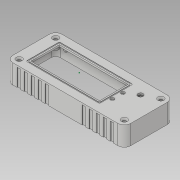
# Autodesk Inventor part: CAJA ELECTRONICA
Saved by Autodesk Inventor 2019 (Build 230136000, 136)
## iProperties
Created: 2020-02-13
Part Number: CAJA ELECTRONICA
Material: Genérico
Document SubType Name: Modeling
Designer: Luis Pujol
Density: 1 g/cm^3
Appearance: Valor por defecto
Author: Luis Pujol
## iProperties of the stored document TAPA SUPERIOR DOSF CO2_3DPrint.ipt
Created: 2020-02-13
Part Number: TAPA SUPERIOR DOSF CO2_3DPrint
Material: Genérico
Document SubType Name: Modeling
Designer: Luis Pujol
Density: 1 g/cm^3
Appearance: Valor por defecto
Author: Luis Pujol
Autodesk Inventor part; units mm, degrees
ref_plane "XZ Plane" through (0, 0, 0) normal (0, 1, 0) x (-1, 0, 0)
ref_plane "XY Plane" through (0, 0, 0) normal (0, 0, 1) x (1, 0, 0)
sketch "Boceto1" plane through (0, 0, 0) normal (0, 1, 0) x (-1, 0, 0)
  line L0 (48.8, 20.25) -> (-48.8, 20.25)
  line L1 (-48.8, 20.25) -> (-48.8, -20.25)
  line L2 (-48.8, -20.25) -> (48.8, -20.25)
  line L3 (48.8, -20.25) -> (48.8, 20.25)
  line L4 (48.8, 20.25) -> (-48.8, -20.25) construction
  line L5 (-48.8, 20.25) -> (48.8, -20.25) construction
  line L6 (-98.8, 35) -> (68.8, 35)
  line L7 (68.8, 35) -> (68.8, -35)
  line L8 (68.8, -35) -> (-98.8, -35)
  line L9 (-98.8, -35) -> (-98.8, 35)
  point P0 (0, 0)
  point P1 (0, 0)
  dimension "d5" = 97.6
  dimension "d6" = 40.5
  dimension "d7" = 70
  dimension "d8" = 20
  dimension "d9" = 50
  constraints: 20 end point, 4 parallel, 3 midpoint, 2 horizontal, 2 perpendicular
  measures "d5" distance of L2.end L1.end
  measures "d6" distance of L1.end L0.end
  measures "d7" distance of L6.end L7.end
  measures "d8" distance between parallel lines of L3 L7
  measures "d9" distance between parallel lines of L1 L9
extrude "Extrusión1" add sketch "Boceto1" along normal blind 2.5
sketch "Boceto2" plane through (0, 0, 0) normal (0, -1, 0) x (1, 0, 0)
  line L0 (-48.8, -20.25) -> (-48.8, 20.25) projected
  line L1 (-48.8, 20.25) -> (48.8, 20.25) projected
  line L2 (48.8, 20.25) -> (48.8, -20.25) projected
  line L3 (48.8, -20.25) -> (-48.8, -20.25) projected
  line L4 (98.8, 35) -> (-68.8, 35) projected
  line L5 (-68.8, 35) -> (-68.8, -35) projected
  line L6 (-68.8, -35) -> (98.8, -35) projected
  line L7 (98.8, -35) -> (98.8, 35) projected
  line L8 (46.5, 27.5) -> (-46.5, 27.5) construction
  line L9 (-46.5, 27.5) -> (-46.5, -27.5) construction
  line L10 (-46.5, -27.5) -> (46.5, -27.5) construction
  line L11 (46.5, -27.5) -> (46.5, 27.5) construction
  line L12 (46.5, 27.5) -> (-46.5, -27.5) construction
  line L13 (-46.5, 27.5) -> (46.5, -27.5) construction
  circle A0 centre (46.5, -27.5) radius 3
  circle A1 centre (-46.5, -27.5) radius 3
  circle A2 centre (46.5, 27.5) radius 3
  circle A3 centre (-46.5, 27.5) radius 3
  point P0 (0, 0)
  dimension "d12" = 93
  dimension "d13" = 55
  dimension "d14" = 6
  dimension "d15" = 6
  dimension "d16" = 6
  dimension "d17" = 6
  constraints: 12 end point, 4 centre point, 4 coincident, 2 midpoint, 2 parallel, 1 horizontal, 1 perpendicular
  measures "d12" distance of L10.end L9.end
  measures "d13" distance of L9.end L8.end
  measures "d14" diameter of A0
  measures "d15" diameter of A1
  measures "d16" diameter of A2
  measures "d17" diameter of A3
extrude "Extrusión2" add sketch "Boceto2" along normal blind 6 contours A0 | A1 | A2 | A3
sketch "Boceto3" plane through (46.5, -6, -27.5) normal (0, -1, 0) x (1, 0, 0)
  circle A0 centre (0, 0) radius 3 projected
  circle A1 centre (-93, 0) radius 3 projected
  circle A2 centre (-93, 55) radius 3 projected
  circle A3 centre (0, 55) radius 3 projected
  circle A4 centre (0, 0) radius 1.5
  circle A5 centre (-93, 0) radius 1.5
  circle A6 centre (-93, 55) radius 1.5
  circle A7 centre (0, 55) radius 1.5
  point P0 (-46.5, 27.5)
  dimension "d20" = 3
  dimension "d21" = 3
  dimension "d22" = 3
  dimension "d23" = 3
  constraints: 4 centre point, 4 coincident
  measures "d20" diameter of A4
  measures "d21" diameter of A5
  measures "d22" diameter of A6
  measures "d23" diameter of A7
extrude "Extrusión3" add sketch "Boceto3" along normal blind 2.5 contours A4 | A5 | A6 | A7
sketch "Boceto4" plane through (0, 2.5, 0) normal (0, 1, 0) x (1, 0, 0)
  line L0 (-48.8, -20.25) -> (-48.8, 20.25) projected
  line L1 (-48.8, 20.25) -> (48.8, 20.25) projected
  line L2 (48.8, 20.25) -> (48.8, -20.25) projected
  line L3 (48.8, -20.25) -> (-48.8, -20.25) projected
  line L4 (-68.8, -35) -> (98.8, -35) projected
  line L5 (98.8, -35) -> (98.8, 35) projected
  line L6 (98.8, 35) -> (-68.8, 35) projected
  line L7 (-68.8, 35) -> (-68.8, -35) projected
  circle A0 centre (70.8, 16) radius 3.65
  circle A1 centre (55.8, 6) radius 2.65
  circle A2 centre (55.8, -9) radius 2.65
  point P0 (0, 0)
  dimension "d26" = 22
  dimension "d27" = 19
  dimension "d28" = 7.3
  dimension "d29" = 15
  dimension "d30" = 10
  dimension "d31" = 15
  dimension "d32" = 5.3
  dimension "d33" = 5.3
  constraints: 3 centre point, 3 coincident, 1 vertical alignment
  measures "d26" distance from line of L2 point (70.8, 16)
  measures "d27" distance from line of L6 point (70.8, 16)
  measures "d28" diameter of A0
  measures "d29" horizontal distance of point (70.8, 16) point (55.8, 6)
  measures "d30" vertical distance of point (70.8, 16) point (55.8, 6)
  measures "d31" distance of point (55.8, 6) point (55.8, -9)
  measures "d32" diameter of A1
  measures "d33" diameter of A2
extrude "Extrusión4" cut sketch "Boceto4" against normal blind 2.5 contours A0 | A1 | A2
fillet "Empalme1" radius 9 4 edges at (-68.8, 1.25, -35) (98.8, 1.25, -35) (-68.8, 1.25, 35) (98.8, 1.25, 35)
sketch "Boceto6" plane through (0, 0, 0) normal (0, -1, 0) x (1, 0, 0)
  circle A0 centre (55.8, 9) radius 2.65 projected
  circle A1 centre (55.8, -6) radius 2.65 projected
  circle A2 centre (70.8, -16) radius 3.65 projected
  circle A3 centre (46.5, 27.5) radius 3 projected
  circle A4 centre (46.5, -27.5) radius 3 projected
  circle A5 centre (-46.5, -27.5) radius 3 projected
  circle A6 centre (-46.5, 27.5) radius 3 projected
  line L0 (-48.8, -20.25) -> (-48.8, 20.25) projected
  line L1 (-48.8, 20.25) -> (48.8, 20.25) projected
  line L2 (48.8, 20.25) -> (48.8, -20.25) projected
  line L3 (48.8, -20.25) -> (-48.8, -20.25) projected
  arc A7 (98.8, 26) -> (89.8, 35) centre (89.8, 26) ccw projected
  line L4 (89.8, 35) -> (-59.8, 35) projected
  arc A8 (-59.8, 35) -> (-68.8, 26) centre (-59.8, 26) ccw projected
  line L5 (-68.8, 26) -> (-68.8, -26) projected
  arc A9 (-68.8, -26) -> (-59.8, -35) centre (-59.8, -26) ccw projected
  line L6 (-59.8, -35) -> (89.8, -35) projected
  arc A10 (89.8, -35) -> (98.8, -26) centre (89.8, -26) ccw projected
  line L7 (98.8, -26) -> (98.8, 26) projected
  line L8 (89.8, -32.5) -> (-59.8, -32.5)
  arc A11 (-66.3, -26) -> (-59.8, -32.5) centre (-59.8, -26) ccw
  line L9 (-66.3, -26) -> (-66.3, 26)
  arc A12 (-59.8, 32.5) -> (-66.3, 26) centre (-59.8, 26) ccw
  line L10 (-59.8, 32.5) -> (89.8, 32.5)
  arc A13 (96.3, 26) -> (89.8, 32.5) centre (89.8, 26) ccw
  line L11 (96.3, 26) -> (96.3, -26)
  arc A14 (89.8, -32.5) -> (96.3, -26) centre (89.8, -26) ccw
  point P0 (0, 0)
  dimension "d37" = 2.5
  constraints: 8 end point, 8 point on circle, 4 centre point, 7 other
  measures "d37" distance between parallel lines of L6 L8
extrude "Extrusión5" add sketch "Boceto6" along normal blind 25 contours L7 A10 L6 A9 L5 A8 L4 A7
sketch "Boceto10" plane through (-59.8, 2.5, 35) normal (0, 0, 1) x (1, 0, 0)
  line L0 (149.6, -27.5) -> (0, -27.5) projected
  line L1 (0, 0) -> (149.6, 0) projected
  line L2 (108.6, -2.5) -> (11, -2.5) projected
  line L3 (11, -27.5) -> (6, -27.5)
  line L4 (6, -27.5) -> (6, -2.5)
  line L5 (6, -2.5) -> (11, -2.5)
  line L6 (11, -2.5) -> (11, -27.5)
  line L7 (-9, 0) -> (-9, -27.5) projected
  point P0 (59.8, -2.5)
  dimension "d53" = 5
  dimension "d54" = 15
  constraints: 8 end point, 2 parallel, 2 point on line, 1 horizontal, 1 perpendicular
  measures "d53" distance of L4.end L5.end
  measures "d54" distance between parallel lines of L7 L4
extrude "Extrusión7" cut sketch "Boceto10" against normal blind 1.2
pattern_linear "Patrón rectangular1" count 5 spacing 10 along (1, 0, 0) of "Extrusión7"
ref_plane "Plano de trabajo1" through (15, 0, 0) normal (1, 0, 0) x (0, 1, 0)
mirror "Simetría1" about plane through (15, 0, 0) normal (1, 0, 0) of "Extrusión7", "Patrón rectangular1"
mirror "Simetría2" about plane through (0, 0, 0) normal (0, 0, 1) of "Extrusión7", "Patrón rectangular1", "Simetría1"
sketch "Boceto12" plane through (0, 2.5, 0) normal (0, 1, 0) x (1, 0, 0)
  point P0 (0, 0)
sketch "Boceto13" plane through (0, 2.5, 0) normal (0, 1, 0) x (1, 0, 0)
  line L0 (89.8, 35) -> (-59.8, 35) projected
  arc A0 (89.8, -35) -> (98.8, -26) centre (89.8, -26) ccw construction
  line L1 (98.8, -26) -> (98.8, 26) construction
  arc A1 (98.8, 26) -> (89.8, 35) centre (89.8, 26) ccw construction
  line L2 (89.8, 35) -> (-59.8, 35) construction
  arc A2 (-59.8, 35) -> (-68.8, 26) centre (-59.8, 26) ccw construction
  line L3 (-68.8, 26) -> (-68.8, -26) construction
  arc A3 (-68.8, -26) -> (-59.8, -35) centre (-59.8, -26) ccw construction
  line L4 (-59.8, -35) -> (89.8, -35) construction
  circle A4 centre (55.8, -9) radius 2.65 construction
  circle A5 centre (55.8, 6) radius 2.65 construction
  circle A6 centre (70.8, 16) radius 3.65 construction
  line L5 (-48.8, -20.25) -> (-48.8, 20.25) construction
  line L6 (-48.8, 20.25) -> (48.8, 20.25) construction
  line L7 (48.8, 20.25) -> (48.8, -20.25) construction
  line L8 (48.8, -20.25) -> (-48.8, -20.25) construction
  line L9 (-59.8, -26) -> (89.8, -26) construction
  line L10 (89.8, -26) -> (89.8, 26) construction
  line L11 (89.8, 26) -> (-59.8, 26) construction
  line L12 (-59.8, 26) -> (-59.8, -26) construction
  line L13 (-59.8, -26) -> (89.8, 26) construction
  line L14 (89.8, -26) -> (-59.8, 26) construction
  point P0 (0, 0)
  point P1 (15, 0)
  constraints: 12 end point, 2 midpoint, 2 parallel, 1 horizontal, 1 perpendicular
hole "Agujero2" at (89.8, 2.5, -26) at (89.8, 2.5, 26) at (-59.8, 2.5, 26) at (-59.8, 2.5, -26) direction (0, -1, 0) diameter 4.5 depth 20 tip angle 118
sketch "Boceto14" plane through (0, 0, 0) normal (0, -1, 0) x (1, 0, 0)
  circle A0 centre (-59.8, 26) radius 2.25 projected
  circle A1 centre (89.8, -26) radius 2.25 projected
  circle A2 centre (89.8, 26) radius 2.25 projected
  circle A3 centre (-59.8, -26) radius 2.25 projected
  arc A4 (-66.3, -26) -> (-59.8, -32.5) centre (-59.8, -26) ccw projected
  line L0 (-59.8, -32.5) -> (89.8, -32.5) projected
  arc A5 (89.8, -32.5) -> (96.3, -26) centre (89.8, -26) ccw projected
  line L1 (96.3, -26) -> (96.3, 26) projected
  arc A6 (96.3, 26) -> (89.8, 32.5) centre (89.8, 26) ccw projected
  line L2 (89.8, 32.5) -> (-59.8, 32.5) projected
  arc A7 (-59.8, 32.5) -> (-66.3, 26) centre (-59.8, 26) ccw projected
  line L3 (-66.3, 26) -> (-66.3, -26) projected
  circle A8 centre (55.8, 9) radius 2.65 projected
  circle A9 centre (55.8, -6) radius 2.65 projected
  circle A10 centre (70.8, -16) radius 3.65 projected
  circle A11 centre (46.5, 27.5) radius 3 projected
  circle A12 centre (46.5, -27.5) radius 3 projected
  circle A13 centre (-46.5, -27.5) radius 3 projected
  circle A14 centre (-46.5, 27.5) radius 3 projected
  line L4 (-48.8, -20.25) -> (-48.8, 20.25) projected
  line L5 (-48.8, 20.25) -> (48.8, 20.25) projected
  line L6 (48.8, 20.25) -> (48.8, -20.25) projected
  line L7 (48.8, -20.25) -> (-48.8, -20.25) projected
  circle A15 centre (89.8, -26) radius 4.25
  circle A16 centre (-59.8, -26) radius 4.25
  circle A17 centre (-59.8, 26) radius 4.25
  circle A18 centre (89.8, 26) radius 4.25
  point P0 (0, 0)
  dimension "d71" = 2
  dimension "d72" = 2
  dimension "d73" = 2
  dimension "d74" = 2
  constraints: 4 centre point
  measures "d71" radial gap between concentric circles of A1 A15
  measures "d72" radial gap between concentric circles of A3 A16
  measures "d73" radial gap between concentric circles of A0 A17
  measures "d74" radial gap between concentric circles of A2 A18
extrude "Extrusión8" add sketch "Boceto14" along normal blind 10 contours A15 | A16 | A17 | A18
chamfer "Chaflán2" distance 2 angle 45 4 edges at (-59.8, 2.5, -28.25) (-59.8, 2.5, 23.75) (89.8, 2.5, -28.25) (89.8, 2.5, 23.75)
sketch "Boceto16" plane through (0, 0, 0) normal (0, -1, 0) x (1, 0, 0)
  line L0 (83.156, 24.1449) -> (83.156, -23.9937) construction
  line L1 (83.156, -23.9937) -> (83.8649, -23.9937) construction
  line L2 (83.8649, -23.9937) -> (83.8649, 24.1449) construction
  line L3 (83.8649, 24.1449) -> (83.156, 24.1449) construction
  line L4 (80.0928, 23.2575) -> (82.5215, 23.2575)
  line L5 (82.5215, 23.2575) -> (82.5215, 24.1449)
  line L6 (82.5215, 24.1449) -> (83.0928, 24.1449)
  line L7 (83.0928, 24.1449) -> (83.0928, 21.6165)
  line L8 (83.0928, 21.6165) -> (82.5215, 21.6165)
  line L9 (82.5215, 21.6165) -> (82.5215, 22.5039)
  line L10 (82.5215, 22.5039) -> (80.0928, 22.5039)
  line L11 (80.0928, 22.5039) -> (80.0928, 23.2575)
  line L12 (80.0928, 21.3078) -> (83.0928, 21.3078)
  line L13 (83.0928, 21.3078) -> (83.0928, 19.2802)
  line L14 (83.0928, 19.2802) -> (82.5215, 19.2802)
  line L15 (82.5215, 19.2802) -> (82.5215, 20.559)
  line L16 (82.5215, 20.559) -> (81.9939, 20.559)
  line L17 (81.9939, 20.559) -> (81.9939, 19.3799)
  line L18 (81.9939, 19.3799) -> (81.4226, 19.3799)
  line L19 (81.4226, 19.3799) -> (81.4226, 20.559)
  line L20 (81.4226, 20.559) -> (80.6641, 20.559)
  line L21 (80.6641, 20.559) -> (80.6641, 19.2802)
  line L22 (80.6641, 19.2802) -> (80.0928, 19.2802)
  line L23 (80.0928, 19.2802) -> (80.0928, 21.3078)
  spline S0 degree 2 poles (80.0344, 17.4763) (80.0344, 18.1522) (80.8513, 18.9447) (81.5904, 18.9447) knots 0 0 0 1 2 2 2
  spline S1 degree 2 poles (81.5904, 18.9447) (82.3027, 18.9447) (83.1511, 18.1497) (83.1511, 17.4739) knots 0 0 0 1 2 2 2
  spline S2 degree 2 poles (83.1511, 17.4739) (83.1511, 17.2964) (83.1098, 17.0095) (83.0758, 16.8783) knots 0 0 0 1 2 2 2
  spline S3 degree 2 poles (83.0758, 16.8783) (83.0442, 16.7762) (82.9396, 16.5355) (82.9007, 16.4601) knots 0 0 0 1 2 2 2
  line L24 (82.9007, 16.4601) -> (82.186, 16.4601)
  line L25 (82.186, 16.4601) -> (82.186, 16.5355)
  spline S4 degree 2 poles (82.186, 16.5355) (82.2346, 16.5914) (82.3707, 16.7567) (82.434, 16.8612) knots 0 0 0 1 2 2 2
  spline S5 degree 2 poles (82.434, 16.8612) (82.4996, 16.9658) (82.5895, 17.2162) (82.5895, 17.3548) knots 0 0 0 1 2 2 2
  spline S6 degree 2 poles (82.5895, 17.3548) (82.5895, 17.5176) (82.4874, 17.7875) (82.3586, 17.9115) knots 0 0 0 1 2 2 2
  spline S7 degree 2 poles (82.3586, 17.9115) (82.2443, 18.0233) (81.8529, 18.1668) (81.5879, 18.1668) knots 0 0 0 1 2 2 2
  spline S8 degree 2 poles (81.5879, 18.1668) (81.3083, 18.1668) (80.9267, 18.0185) (80.81, 17.8969) knots 0 0 0 1 2 2 2
  spline S9 degree 2 poles (80.81, 17.8969) (80.6957, 17.7802) (80.596, 17.4933) (80.596, 17.3499) knots 0 0 0 1 2 2 2
  spline S10 degree 2 poles (80.596, 17.3499) (80.596, 17.2016) (80.6957, 16.9317) (80.7565, 16.8394) knots 0 0 0 1 2 2 2
  spline S11 degree 2 poles (80.7565, 16.8394) (80.8173, 16.7373) (80.9461, 16.5841) (80.9972, 16.5282) knots 0 0 0 1 2 2 2
  line L26 (80.9972, 16.5282) -> (80.9972, 16.4601)
  line L27 (80.9972, 16.4601) -> (80.2921, 16.4601)
  spline S12 degree 2 poles (80.2921, 16.4601) (80.2532, 16.5428) (80.156, 16.7591) (80.122, 16.8758) knots 0 0 0 1 2 2 2
  spline S13 degree 2 poles (80.122, 16.8758) (80.0782, 17.0168) (80.0344, 17.2624) (80.0344, 17.4763) knots 0 0 0 1 2 2 2
  line L28 (80.0928, 13.4455) -> (80.0928, 14.17)
  line L29 (80.0928, 14.17) -> (82.1835, 15.3272)
  line L30 (82.1835, 15.3272) -> (80.0928, 15.3272)
  line L31 (80.0928, 15.3272) -> (80.0928, 16.0152)
  line L32 (80.0928, 16.0152) -> (83.0928, 16.0152)
  line L33 (83.0928, 16.0152) -> (83.0928, 15.0914)
  line L34 (83.0928, 15.0914) -> (81.374, 14.1335)
  line L35 (81.374, 14.1335) -> (83.0928, 14.1335)
  line L36 (83.0928, 14.1335) -> (83.0928, 13.4455)
  line L37 (83.0928, 13.4455) -> (80.0928, 13.4455)
  spline S14 degree 2 poles (81.5928, 10.1052) (80.8635, 10.1052) (80.0296, 10.8831) (80.0296, 11.559) knots 0 0 0 1 2 2 2
  spline S15 degree 2 poles (80.0296, 11.559) (80.0296, 12.2373) (80.8732, 13.0104) (81.5928, 13.0104) knots 0 0 0 1 2 2 2
  spline S16 degree 2 poles (81.5928, 13.0104) (82.3148, 13.0104) (83.156, 12.2373) (83.156, 11.559) knots 0 0 0 1 2 2 2
  spline S17 degree 2 poles (83.156, 11.559) (83.156, 10.8831) (82.3197, 10.1052) (81.5928, 10.1052) knots 0 0 0 1 2 2 2
  spline S18 degree 2 poles (81.5928, 10.8831) (81.8626, 10.8831) (82.2395, 10.9925) (82.3586, 11.0873) knots 0 0 0 1 2 2 2
  spline S19 degree 2 poles (82.3586, 11.0873) (82.4826, 11.1822) (82.5895, 11.4253) (82.5895, 11.5565) knots 0 0 0 1 2 2 2
  spline S20 degree 2 poles (82.5895, 11.5565) (82.5895, 11.6951) (82.4899, 11.9212) (82.3635, 12.0258) knots 0 0 0 1 2 2 2
  spline S21 degree 2 poles (82.3635, 12.0258) (82.2468, 12.1181) (81.8602, 12.2324) (81.5928, 12.2324) knots 0 0 0 1 2 2 2
  spline S22 degree 2 poles (81.5928, 12.2324) (81.3156, 12.2324) (80.951, 12.123) (80.827, 12.0282) knots 0 0 0 1 2 2 2
  spline S23 degree 2 poles (80.827, 12.0282) (80.703, 11.9334) (80.596, 11.6878) (80.596, 11.5565) knots 0 0 0 1 2 2 2
  spline S24 degree 2 poles (80.596, 11.5565) (80.596, 11.4228) (80.7103, 11.1749) (80.8318, 11.0849) knots 0 0 0 1 2 2 2
  spline S25 degree 2 poles (80.8318, 11.0849) (80.9631, 10.9877) (81.3108, 10.8831) (81.5928, 10.8831) knots 0 0 0 1 2 2 2
  spline S26 degree 2 poles (80.0344, 8.3645) (80.0344, 9.0403) (80.8513, 9.8329) (81.5904, 9.8329) knots 0 0 0 1 2 2 2
  spline S27 degree 2 poles (81.5904, 9.8329) (82.3027, 9.8329) (83.1511, 9.0379) (83.1511, 8.3621) knots 0 0 0 1 2 2 2
  spline S28 degree 2 poles (83.1511, 8.3621) (83.1511, 8.1846) (83.1098, 7.8977) (83.0758, 7.7664) knots 0 0 0 1 2 2 2
  spline S29 degree 2 poles (83.0758, 7.7664) (83.0442, 7.6643) (82.9396, 7.4236) (82.9007, 7.3483) knots 0 0 0 1 2 2 2
  line L38 (82.9007, 7.3483) -> (82.186, 7.3483)
  line L39 (82.186, 7.3483) -> (82.186, 7.4236)
  spline S30 degree 2 poles (82.186, 7.4236) (82.2346, 7.4796) (82.3707, 7.6449) (82.434, 7.7494) knots 0 0 0 1 2 2 2
  spline S31 degree 2 poles (82.434, 7.7494) (82.4996, 7.854) (82.5895, 8.1044) (82.5895, 8.2429) knots 0 0 0 1 2 2 2
  spline S32 degree 2 poles (82.5895, 8.2429) (82.5895, 8.4058) (82.4874, 8.6757) (82.3586, 8.7997) knots 0 0 0 1 2 2 2
  spline S33 degree 2 poles (82.3586, 8.7997) (82.2443, 8.9115) (81.8529, 9.0549) (81.5879, 9.0549) knots 0 0 0 1 2 2 2
  spline S34 degree 2 poles (81.5879, 9.0549) (81.3083, 9.0549) (80.9267, 8.9066) (80.81, 8.7851) knots 0 0 0 1 2 2 2
  spline S35 degree 2 poles (80.81, 8.7851) (80.6957, 8.6684) (80.596, 8.3815) (80.596, 8.2381) knots 0 0 0 1 2 2 2
  spline S36 degree 2 poles (80.596, 8.2381) (80.596, 8.0898) (80.6957, 7.8199) (80.7565, 7.7275) knots 0 0 0 1 2 2 2
  spline S37 degree 2 poles (80.7565, 7.7275) (80.8173, 7.6254) (80.9461, 7.4723) (80.9972, 7.4164) knots 0 0 0 1 2 2 2
  line L40 (80.9972, 7.4164) -> (80.9972, 7.3483)
  line L41 (80.9972, 7.3483) -> (80.2921, 7.3483)
  spline S38 degree 2 poles (80.2921, 7.3483) (80.2532, 7.4309) (80.156, 7.6473) (80.122, 7.764) knots 0 0 0 1 2 2 2
  spline S39 degree 2 poles (80.122, 7.764) (80.0782, 7.905) (80.0344, 8.1505) (80.0344, 8.3645) knots 0 0 0 1 2 2 2
  spline S40 degree 2 poles (81.5928, 4.1732) (80.8635, 4.1732) (80.0296, 4.9512) (80.0296, 5.627) knots 0 0 0 1 2 2 2
  spline S41 degree 2 poles (80.0296, 5.627) (80.0296, 6.3053) (80.8732, 7.0784) (81.5928, 7.0784) knots 0 0 0 1 2 2 2
  spline S42 degree 2 poles (81.5928, 7.0784) (82.3148, 7.0784) (83.156, 6.3053) (83.156, 5.627) knots 0 0 0 1 2 2 2
  spline S43 degree 2 poles (83.156, 5.627) (83.156, 4.9512) (82.3197, 4.1732) (81.5928, 4.1732) knots 0 0 0 1 2 2 2
  spline S44 degree 2 poles (81.5928, 4.9512) (81.8626, 4.9512) (82.2395, 5.0606) (82.3586, 5.1554) knots 0 0 0 1 2 2 2
  spline S45 degree 2 poles (82.3586, 5.1554) (82.4826, 5.2502) (82.5895, 5.4933) (82.5895, 5.6246) knots 0 0 0 1 2 2 2
  spline S46 degree 2 poles (82.5895, 5.6246) (82.5895, 5.7632) (82.4899, 5.9893) (82.3635, 6.0938) knots 0 0 0 1 2 2 2
  spline S47 degree 2 poles (82.3635, 6.0938) (82.2468, 6.1862) (81.8602, 6.3005) (81.5928, 6.3005) knots 0 0 0 1 2 2 2
  spline S48 degree 2 poles (81.5928, 6.3005) (81.3156, 6.3005) (80.951, 6.1911) (80.827, 6.0963) knots 0 0 0 1 2 2 2
  spline S49 degree 2 poles (80.827, 6.0963) (80.703, 6.0014) (80.596, 5.7559) (80.596, 5.6246) knots 0 0 0 1 2 2 2
  spline S50 degree 2 poles (80.596, 5.6246) (80.596, 5.4909) (80.7103, 5.2429) (80.8318, 5.153) knots 0 0 0 1 2 2 2
  spline S51 degree 2 poles (80.8318, 5.153) (80.9631, 5.0557) (81.3108, 4.9512) (81.5928, 4.9512) knots 0 0 0 1 2 2 2
  line L42 (80.0928, 1.1562) -> (80.0928, 1.8807)
  line L43 (80.0928, 1.8807) -> (82.1835, 3.0379)
  line L44 (82.1835, 3.0379) -> (80.0928, 3.0379)
  line L45 (80.0928, 3.0379) -> (80.0928, 3.7259)
  line L46 (80.0928, 3.7259) -> (83.0928, 3.7259)
  line L47 (83.0928, 3.7259) -> (83.0928, 2.8021)
  line L48 (83.0928, 2.8021) -> (81.374, 1.8442)
  line L49 (81.374, 1.8442) -> (83.0928, 1.8442)
  line L50 (83.0928, 1.8442) -> (83.0928, 1.1562)
  line L51 (83.0928, 1.1562) -> (80.0928, 1.1562)
  spline S52 degree 2 poles (80.0344, -0.7473) (80.0344, -0.0715) (80.8513, 0.7211) (81.5904, 0.7211) knots 0 0 0 1 2 2 2
  spline S53 degree 2 poles (81.5904, 0.7211) (82.3027, 0.7211) (83.1511, -0.0739) (83.1511, -0.7498) knots 0 0 0 1 2 2 2
  spline S54 degree 2 poles (83.1511, -0.7498) (83.1511, -0.9272) (83.1098, -1.2141) (83.0758, -1.3454) knots 0 0 0 1 2 2 2
  spline S55 degree 2 poles (83.0758, -1.3454) (83.0442, -1.4475) (82.9396, -1.6882) (82.9007, -1.7636) knots 0 0 0 1 2 2 2
  line L52 (82.9007, -1.7636) -> (82.186, -1.7636)
  line L53 (82.186, -1.7636) -> (82.186, -1.6882)
  spline S56 degree 2 poles (82.186, -1.6882) (82.2346, -1.6323) (82.3707, -1.467) (82.434, -1.3624) knots 0 0 0 1 2 2 2
  spline S57 degree 2 poles (82.434, -1.3624) (82.4996, -1.2579) (82.5895, -1.0075) (82.5895, -0.8689) knots 0 0 0 1 2 2 2
  spline S58 degree 2 poles (82.5895, -0.8689) (82.5895, -0.706) (82.4874, -0.4362) (82.3586, -0.3122) knots 0 0 0 1 2 2 2
  spline S59 degree 2 poles (82.3586, -0.3122) (82.2443, -0.2003) (81.8529, -0.0569) (81.5879, -0.0569) knots 0 0 0 1 2 2 2
  spline S60 degree 2 poles (81.5879, -0.0569) (81.3083, -0.0569) (80.9267, -0.2052) (80.81, -0.3268) knots 0 0 0 1 2 2 2
  spline S61 degree 2 poles (80.81, -0.3268) (80.6957, -0.4435) (80.596, -0.7303) (80.596, -0.8738) knots 0 0 0 1 2 2 2
  spline S62 degree 2 poles (80.596, -0.8738) (80.596, -1.0221) (80.6957, -1.2919) (80.7565, -1.3843) knots 0 0 0 1 2 2 2
  spline S63 degree 2 poles (80.7565, -1.3843) (80.8173, -1.4864) (80.9461, -1.6396) (80.9972, -1.6955) knots 0 0 0 1 2 2 2
  line L54 (80.9972, -1.6955) -> (80.9972, -1.7636)
  line L55 (80.9972, -1.7636) -> (80.2921, -1.7636)
  spline S64 degree 2 poles (80.2921, -1.7636) (80.2532, -1.6809) (80.156, -1.4645) (80.122, -1.3478) knots 0 0 0 1 2 2 2
  spline S65 degree 2 poles (80.122, -1.3478) (80.0782, -1.2068) (80.0344, -0.9613) (80.0344, -0.7473) knots 0 0 0 1 2 2 2
  line L56 (80.0928, -3.7012) -> (80.0928, -2.0869)
  line L57 (80.0928, -2.0869) -> (80.6155, -2.0869)
  line L58 (80.6155, -2.0869) -> (80.6155, -2.5172)
  line L59 (80.6155, -2.5172) -> (82.5701, -2.5172)
  line L60 (82.5701, -2.5172) -> (82.5701, -2.0869)
  line L61 (82.5701, -2.0869) -> (83.0928, -2.0869)
  line L62 (83.0928, -2.0869) -> (83.0928, -3.7012)
  line L63 (83.0928, -3.7012) -> (82.5701, -3.7012)
  line L64 (82.5701, -3.7012) -> (82.5701, -3.2708)
  line L65 (82.5701, -3.2708) -> (80.6155, -3.2708)
  line L66 (80.6155, -3.2708) -> (80.6155, -3.7012)
  line L67 (80.6155, -3.7012) -> (80.0928, -3.7012)
  line L68 (80.0928, -4.202) -> (83.0928, -4.202)
  line L69 (83.0928, -4.202) -> (83.0928, -6.2295)
  line L70 (83.0928, -6.2295) -> (82.5215, -6.2295)
  line L71 (82.5215, -6.2295) -> (82.5215, -4.9507)
  line L72 (82.5215, -4.9507) -> (81.9939, -4.9507)
  line L73 (81.9939, -4.9507) -> (81.9939, -6.1298)
  line L74 (81.9939, -6.1298) -> (81.4226, -6.1298)
  line L75 (81.4226, -6.1298) -> (81.4226, -4.9507)
  line L76 (81.4226, -4.9507) -> (80.6641, -4.9507)
  line L77 (80.6641, -4.9507) -> (80.6641, -6.2295)
  line L78 (80.6641, -6.2295) -> (80.0928, -6.2295)
  line L79 (80.0928, -6.2295) -> (80.0928, -4.202)
  line L80 (80.0928, -9.3097) -> (80.0928, -8.5853)
  line L81 (80.0928, -8.5853) -> (82.1835, -7.4281)
  line L82 (82.1835, -7.4281) -> (80.0928, -7.4281)
  line L83 (80.0928, -7.4281) -> (80.0928, -6.7401)
  line L84 (80.0928, -6.7401) -> (83.0928, -6.7401)
  line L85 (83.0928, -6.7401) -> (83.0928, -7.6639)
  line L86 (83.0928, -7.6639) -> (81.374, -8.6217)
  line L87 (81.374, -8.6217) -> (83.0928, -8.6217)
  line L88 (83.0928, -8.6217) -> (83.0928, -9.3097)
  line L89 (83.0928, -9.3097) -> (80.0928, -9.3097)
  spline S66 degree 2 poles (80.0344, -11.2133) (80.0344, -10.5375) (80.8513, -9.7449) (81.5904, -9.7449) knots 0 0 0 1 2 2 2
  spline S67 degree 2 poles (81.5904, -9.7449) (82.3027, -9.7449) (83.1511, -10.5399) (83.1511, -11.2157) knots 0 0 0 1 2 2 2
  spline S68 degree 2 poles (83.1511, -11.2157) (83.1511, -11.3932) (83.1098, -11.6801) (83.0758, -11.8114) knots 0 0 0 1 2 2 2
  spline S69 degree 2 poles (83.0758, -11.8114) (83.0442, -11.9135) (82.9396, -12.1542) (82.9007, -12.2295) knots 0 0 0 1 2 2 2
  line L90 (82.9007, -12.2295) -> (82.186, -12.2295)
  line L91 (82.186, -12.2295) -> (82.186, -12.1542)
  spline S70 degree 2 poles (82.186, -12.1542) (82.2346, -12.0982) (82.3707, -11.9329) (82.434, -11.8284) knots 0 0 0 1 2 2 2
  spline S71 degree 2 poles (82.434, -11.8284) (82.4996, -11.7238) (82.5895, -11.4734) (82.5895, -11.3349) knots 0 0 0 1 2 2 2
  spline S72 degree 2 poles (82.5895, -11.3349) (82.5895, -11.172) (82.4874, -10.9021) (82.3586, -10.7781) knots 0 0 0 1 2 2 2
  spline S73 degree 2 poles (82.3586, -10.7781) (82.2443, -10.6663) (81.8529, -10.5229) (81.5879, -10.5229) knots 0 0 0 1 2 2 2
  spline S74 degree 2 poles (81.5879, -10.5229) (81.3083, -10.5229) (80.9267, -10.6712) (80.81, -10.7927) knots 0 0 0 1 2 2 2
  spline S75 degree 2 poles (80.81, -10.7927) (80.6957, -10.9094) (80.596, -11.1963) (80.596, -11.3397) knots 0 0 0 1 2 2 2
  spline S76 degree 2 poles (80.596, -11.3397) (80.596, -11.488) (80.6957, -11.7579) (80.7565, -11.8503) knots 0 0 0 1 2 2 2
  spline S77 degree 2 poles (80.7565, -11.8503) (80.8173, -11.9524) (80.9461, -12.1055) (80.9972, -12.1614) knots 0 0 0 1 2 2 2
  line L92 (80.9972, -12.1614) -> (80.9972, -12.2295)
  line L93 (80.9972, -12.2295) -> (80.2921, -12.2295)
  spline S78 degree 2 poles (80.2921, -12.2295) (80.2532, -12.1469) (80.156, -11.9305) (80.122, -11.8138) knots 0 0 0 1 2 2 2
  spline S79 degree 2 poles (80.122, -11.8138) (80.0782, -11.6728) (80.0344, -11.4272) (80.0344, -11.2133) knots 0 0 0 1 2 2 2
  line L94 (80.0928, -14.1671) -> (80.0928, -12.5529)
  line L95 (80.0928, -12.5529) -> (80.6155, -12.5529)
  line L96 (80.6155, -12.5529) -> (80.6155, -12.9832)
  line L97 (80.6155, -12.9832) -> (82.5701, -12.9832)
  line L98 (82.5701, -12.9832) -> (82.5701, -12.5529)
  line L99 (82.5701, -12.5529) -> (83.0928, -12.5529)
  line L100 (83.0928, -12.5529) -> (83.0928, -14.1671)
  line L101 (83.0928, -14.1671) -> (82.5701, -14.1671)
  line L102 (82.5701, -14.1671) -> (82.5701, -13.7368)
  line L103 (82.5701, -13.7368) -> (80.6155, -13.7368)
  line L104 (80.6155, -13.7368) -> (80.6155, -14.1671)
  line L105 (80.6155, -14.1671) -> (80.0928, -14.1671)
  line L106 (80.0928, -14.3446) -> (83.0928, -15.3584)
  line L107 (83.0928, -15.3584) -> (83.0928, -16.1801)
  line L108 (83.0928, -16.1801) -> (80.0928, -17.1939)
  line L109 (80.0928, -17.1939) -> (80.0928, -16.4183)
  line L110 (80.0928, -16.4183) -> (80.7054, -16.2311)
  line L111 (80.7054, -16.2311) -> (80.7054, -15.2879)
  line L112 (80.7054, -15.2879) -> (80.0928, -15.0982)
  line L113 (80.0928, -15.0982) -> (80.0928, -14.3446)
  line L114 (81.25, -16.0658) -> (82.2419, -15.7595)
  line L115 (82.2419, -15.7595) -> (81.25, -15.4507)
  line L116 (81.25, -15.4507) -> (81.25, -16.0658)
  spline S80 degree 2 poles (80.0344, -19.9945) (80.0344, -19.3187) (80.8513, -18.5261) (81.5904, -18.5261) knots 0 0 0 1 2 2 2
  spline S81 degree 2 poles (81.5904, -18.5261) (82.3027, -18.5261) (83.1511, -19.3211) (83.1511, -19.9969) knots 0 0 0 1 2 2 2
  spline S82 degree 2 poles (83.1511, -19.9969) (83.1511, -20.1744) (83.1098, -20.4613) (83.0758, -20.5926) knots 0 0 0 1 2 2 2
  spline S83 degree 2 poles (83.0758, -20.5926) (83.0442, -20.6947) (82.9396, -20.9354) (82.9007, -21.0107) knots 0 0 0 1 2 2 2
  line L117 (82.9007, -21.0107) -> (82.186, -21.0107)
  line L118 (82.186, -21.0107) -> (82.186, -20.9354)
  spline S84 degree 2 poles (82.186, -20.9354) (82.2346, -20.8794) (82.3707, -20.7141) (82.434, -20.6096) knots 0 0 0 1 2 2 2
  spline S85 degree 2 poles (82.434, -20.6096) (82.4996, -20.505) (82.5895, -20.2546) (82.5895, -20.1161) knots 0 0 0 1 2 2 2
  spline S86 degree 2 poles (82.5895, -20.1161) (82.5895, -19.9532) (82.4874, -19.6833) (82.3586, -19.5593) knots 0 0 0 1 2 2 2
  spline S87 degree 2 poles (82.3586, -19.5593) (82.2443, -19.4475) (81.8529, -19.3041) (81.5879, -19.3041) knots 0 0 0 1 2 2 2
  spline S88 degree 2 poles (81.5879, -19.3041) (81.3083, -19.3041) (80.9267, -19.4524) (80.81, -19.5739) knots 0 0 0 1 2 2 2
  spline S89 degree 2 poles (80.81, -19.5739) (80.6957, -19.6906) (80.596, -19.9775) (80.596, -20.1209) knots 0 0 0 1 2 2 2
  spline S90 degree 2 poles (80.596, -20.1209) (80.596, -20.2692) (80.6957, -20.5391) (80.7565, -20.6315) knots 0 0 0 1 2 2 2
  spline S91 degree 2 poles (80.7565, -20.6315) (80.8173, -20.7336) (80.9461, -20.8867) (80.9972, -20.9426) knots 0 0 0 1 2 2 2
  line L119 (80.9972, -20.9426) -> (80.9972, -21.0107)
  line L120 (80.9972, -21.0107) -> (80.2921, -21.0107)
  spline S92 degree 2 poles (80.2921, -21.0107) (80.2532, -20.9281) (80.156, -20.7117) (80.122, -20.595) knots 0 0 0 1 2 2 2
  spline S93 degree 2 poles (80.122, -20.595) (80.0782, -20.454) (80.0344, -20.2084) (80.0344, -19.9945) knots 0 0 0 1 2 2 2
  line L121 (80.0928, -21.1323) -> (83.0928, -22.146)
  line L122 (83.0928, -22.146) -> (83.0928, -22.9678)
  line L123 (83.0928, -22.9678) -> (80.0928, -23.9815)
  line L124 (80.0928, -23.9815) -> (80.0928, -23.206)
  line L125 (80.0928, -23.206) -> (80.7054, -23.0188)
  line L126 (80.7054, -23.0188) -> (80.7054, -22.0755)
  line L127 (80.7054, -22.0755) -> (80.0928, -21.8859)
  line L128 (80.0928, -21.8859) -> (80.0928, -21.1323)
  line L129 (81.25, -22.8535) -> (82.2419, -22.5472)
  line L130 (82.2419, -22.5472) -> (81.25, -22.2384)
  line L131 (81.25, -22.2384) -> (81.25, -22.8535)
  point P0 (0, 0)
  constraints: 2 other
extrude "Extrusión10" add sketch "Boceto16" along normal blind 1.5
chamfer "Chaflán3" distance 1.5 angle 45 8 edges at (85.55, 0, 26) (85.55, 0, -26) (-64.05, 0, -26) (-64.05, 0, 26) (-49.5, 0, 27.5) (43.5, 0, 27.5) (43.5, 0, -27.5) (-49.5, 0, -27.5)
sketch "Boceto18" plane through (0, 2.5, 0) normal (0, 1, 0) x (1, 0, 0)
  circle A0 centre (89.8, 26) radius 4.25 projected
  circle A1 centre (-59.8, 26) radius 4.25 projected
  arc A2 (89.8, -35) -> (98.8, -26) centre (89.8, -26) ccw projected
  line L0 (98.8, -26) -> (98.8, 26) projected
  arc A3 (98.8, 26) -> (89.8, 35) centre (89.8, 26) ccw projected
  line L1 (89.8, 35) -> (-59.8, 35) projected
  arc A4 (-59.8, 35) -> (-68.8, 26) centre (-59.8, 26) ccw projected
  line L2 (-68.8, 26) -> (-68.8, -26) projected
  arc A5 (-68.8, -26) -> (-59.8, -35) centre (-59.8, -26) ccw projected
  line L3 (-59.8, -35) -> (89.8, -35) projected
  circle A6 centre (55.8, -9) radius 2.65 projected
  circle A7 centre (55.8, 6) radius 2.65 projected
  circle A8 centre (70.8, 16) radius 3.65 projected
  line L4 (-48.8, -20.25) -> (-48.8, 20.25) projected
  line L5 (-48.8, 20.25) -> (48.8, 20.25) projected
  line L6 (48.8, 20.25) -> (48.8, -20.25) projected
  line L7 (48.8, -20.25) -> (-48.8, -20.25) projected
  circle A9 centre (-59.8, -26) radius 4.25 projected
  circle A10 centre (89.8, -26) radius 4.25 projected
  line L8 (50.8, 22.25) -> (-50.8, 22.25)
  line L9 (-50.8, 22.25) -> (-50.8, -22.25)
  line L10 (-50.8, -22.25) -> (50.8, -22.25)
  line L11 (50.8, -22.25) -> (50.8, 22.25)
  line L12 (-52.3, 23.75) -> (52.3, 23.75)
  line L13 (52.3, 23.75) -> (52.3, -23.75)
  line L14 (52.3, -23.75) -> (-52.3, -23.75)
  line L15 (-52.3, -23.75) -> (-52.3, 23.75)
  point P0 (0, 0)
  dimension "d93" = 2
  dimension "d94" = 1.5
  constraints: 16 end point, 6 other
  measures "d93" distance between parallel lines of L5 L8
  measures "d94" distance between parallel lines of L8 L12
extrude "Extrusión11" cut sketch "Boceto18" against normal blind 0.5 contours L12 L13 L14 L15
fillet "Empalme2" radius 2 8 edges at (52.3, 2.25, -23.75) (50.8, 2.25, -22.25) (52.3, 2.25, 23.75) (50.8, 2.25, 22.25) (-52.3, 2.25, 23.75) (-50.8, 2.25, 22.25) (-52.3, 2.25, -23.75) (-50.8, 2.25, -22.25)
sketch "Boceto19" plane through (0, 0, 0) normal (0, -1, 0) x (1, 0, 0)
  circle A0 centre (46.5, -27.5) radius 4.5 projected
  circle A1 centre (-46.5, 27.5) radius 4.5 projected
  circle A2 centre (-59.8, -26) radius 5.75 projected
  circle A3 centre (89.8, 26) radius 5.75 projected
  line L0 (83.0928, -22.146) -> (83.0928, -22.9678) projected
  line L1 (83.0928, -22.9678) -> (80.0928, -23.9815) projected
  line L2 (80.0928, -23.9815) -> (80.0928, -23.206) projected
  line L3 (80.0928, -23.206) -> (80.7054, -23.0188) projected
  line L4 (80.7054, -23.0188) -> (80.7054, -22.0755) projected
  line L5 (80.7054, -22.0755) -> (80.0928, -21.8859) projected
  line L6 (80.0928, -21.8859) -> (80.0928, -21.1323) projected
  line L7 (80.0928, -21.1323) -> (83.0928, -22.146) projected
  line L8 (80.0928, -12.5529) -> (80.6155, -12.5529) projected
  line L9 (80.6155, -12.5529) -> (80.6155, -12.9832) projected
  line L10 (80.6155, -12.9832) -> (82.5701, -12.9832) projected
  line L11 (82.5701, -12.9832) -> (82.5701, -12.5529) projected
  line L12 (82.5701, -12.5529) -> (83.0928, -12.5529) projected
  line L13 (83.0928, -12.5529) -> (83.0928, -14.1671) projected
  line L14 (83.0928, -14.1671) -> (82.5701, -14.1671) projected
  line L15 (82.5701, -14.1671) -> (82.5701, -13.7368) projected
  line L16 (82.5701, -13.7368) -> (80.6155, -13.7368) projected
  line L17 (80.6155, -13.7368) -> (80.6155, -14.1671) projected
  line L18 (80.6155, -14.1671) -> (80.0928, -14.1671) projected
  line L19 (80.0928, -14.1671) -> (80.0928, -12.5529) projected
  line L20 (80.0928, -8.5853) -> (82.1835, -7.4281) projected
  line L21 (82.1835, -7.4281) -> (80.0928, -7.4281) projected
  line L22 (80.0928, -7.4281) -> (80.0928, -6.7401) projected
  line L23 (80.0928, -6.7401) -> (83.0928, -6.7401) projected
  line L24 (83.0928, -6.7401) -> (83.0928, -7.6639) projected
  line L25 (83.0928, -7.6639) -> (81.374, -8.6217) projected
  line L26 (81.374, -8.6217) -> (83.0928, -8.6217) projected
  line L27 (83.0928, -8.6217) -> (83.0928, -9.3097) projected
  line L28 (83.0928, -9.3097) -> (80.0928, -9.3097) projected
  line L29 (80.0928, -9.3097) -> (80.0928, -8.5853) projected
  line L30 (80.0928, -2.0869) -> (80.6155, -2.0869) projected
  line L31 (80.6155, -2.0869) -> (80.6155, -2.5172) projected
  line L32 (80.6155, -2.5172) -> (82.5701, -2.5172) projected
  line L33 (82.5701, -2.5172) -> (82.5701, -2.0869) projected
  line L34 (82.5701, -2.0869) -> (83.0928, -2.0869) projected
  line L35 (83.0928, -2.0869) -> (83.0928, -3.7012) projected
  line L36 (83.0928, -3.7012) -> (82.5701, -3.7012) projected
  line L37 (82.5701, -3.7012) -> (82.5701, -3.2708) projected
  line L38 (82.5701, -3.2708) -> (80.6155, -3.2708) projected
  line L39 (80.6155, -3.2708) -> (80.6155, -3.7012) projected
  line L40 (80.6155, -3.7012) -> (80.0928, -3.7012) projected
  line L41 (80.0928, -3.7012) -> (80.0928, -2.0869) projected
  line L42 (80.0928, 1.8807) -> (82.1835, 3.0379) projected
  line L43 (82.1835, 3.0379) -> (80.0928, 3.0379) projected
  line L44 (80.0928, 3.0379) -> (80.0928, 3.7259) projected
  line L45 (80.0928, 3.7259) -> (83.0928, 3.7259) projected
  line L46 (83.0928, 3.7259) -> (83.0928, 2.8021) projected
  line L47 (83.0928, 2.8021) -> (81.374, 1.8442) projected
  line L48 (81.374, 1.8442) -> (83.0928, 1.8442) projected
  line L49 (83.0928, 1.8442) -> (83.0928, 1.1562) projected
  line L50 (83.0928, 1.1562) -> (80.0928, 1.1562) projected
  line L51 (80.0928, 1.1562) -> (80.0928, 1.8807) projected
  line L52 (80.0928, 14.17) -> (82.1835, 15.3272) projected
  line L53 (82.1835, 15.3272) -> (80.0928, 15.3272) projected
  line L54 (80.0928, 15.3272) -> (80.0928, 16.0152) projected
  line L55 (80.0928, 16.0152) -> (83.0928, 16.0152) projected
  line L56 (83.0928, 16.0152) -> (83.0928, 15.0914) projected
  line L57 (83.0928, 15.0914) -> (81.374, 14.1335) projected
  line L58 (81.374, 14.1335) -> (83.0928, 14.1335) projected
  line L59 (83.0928, 14.1335) -> (83.0928, 13.4455) projected
  line L60 (83.0928, 13.4455) -> (80.0928, 13.4455) projected
  line L61 (80.0928, 13.4455) -> (80.0928, 14.17) projected
  line L62 (83.0928, 21.3078) -> (83.0928, 19.2802) projected
  line L63 (83.0928, 19.2802) -> (82.5215, 19.2802) projected
  line L64 (82.5215, 19.2802) -> (82.5215, 20.559) projected
  line L65 (82.5215, 20.559) -> (81.9939, 20.559) projected
  line L66 (81.9939, 20.559) -> (81.9939, 19.3799) projected
  line L67 (81.9939, 19.3799) -> (81.4226, 19.3799) projected
  line L68 (81.4226, 19.3799) -> (81.4226, 20.559) projected
  line L69 (81.4226, 20.559) -> (80.6641, 20.559) projected
  line L70 (80.6641, 20.559) -> (80.6641, 19.2802) projected
  line L71 (80.6641, 19.2802) -> (80.0928, 19.2802) projected
  line L72 (80.0928, 19.2802) -> (80.0928, 21.3078) projected
  line L73 (80.0928, 21.3078) -> (83.0928, 21.3078) projected
  line L74 (82.5215, 23.2575) -> (82.5215, 24.1449) projected
  line L75 (82.5215, 24.1449) -> (83.0928, 24.1449) projected
  line L76 (83.0928, 24.1449) -> (83.0928, 21.6165) projected
  line L77 (83.0928, 21.6165) -> (82.5215, 21.6165) projected
  line L78 (82.5215, 21.6165) -> (82.5215, 22.5039) projected
  line L79 (82.5215, 22.5039) -> (80.0928, 22.5039) projected
  line L80 (80.0928, 22.5039) -> (80.0928, 23.2575) projected
  line L81 (80.0928, 23.2575) -> (82.5215, 23.2575) projected
  line L82 (82.9007, 16.4601) -> (82.186, 16.4601) projected
  line L83 (82.186, 16.4601) -> (82.186, 16.5355) projected
  line L84 (80.9972, 16.5282) -> (80.9972, 16.4601) projected
  line L85 (80.9972, 16.4601) -> (80.2921, 16.4601) projected
  line L86 (82.9007, 7.3483) -> (82.186, 7.3483) projected
  line L87 (82.186, 7.3483) -> (82.186, 7.4236) projected
  line L88 (80.9972, 7.4164) -> (80.9972, 7.3483) projected
  line L89 (80.9972, 7.3483) -> (80.2921, 7.3483) projected
  line L90 (82.9007, -1.7636) -> (82.186, -1.7636) projected
  line L91 (82.186, -1.7636) -> (82.186, -1.6882) projected
  line L92 (80.9972, -1.6955) -> (80.9972, -1.7636) projected
  line L93 (80.9972, -1.7636) -> (80.2921, -1.7636) projected
  line L94 (83.0928, -4.202) -> (83.0928, -6.2295) projected
  line L95 (83.0928, -6.2295) -> (82.5215, -6.2295) projected
  line L96 (82.5215, -6.2295) -> (82.5215, -4.9507) projected
  line L97 (82.5215, -4.9507) -> (81.9939, -4.9507) projected
  line L98 (81.9939, -4.9507) -> (81.9939, -6.1298) projected
  line L99 (81.9939, -6.1298) -> (81.4226, -6.1298) projected
  line L100 (81.4226, -6.1298) -> (81.4226, -4.9507) projected
  line L101 (81.4226, -4.9507) -> (80.6641, -4.9507) projected
  line L102 (80.6641, -4.9507) -> (80.6641, -6.2295) projected
  line L103 (80.6641, -6.2295) -> (80.0928, -6.2295) projected
  line L104 (80.0928, -6.2295) -> (80.0928, -4.202) projected
  line L105 (80.0928, -4.202) -> (83.0928, -4.202) projected
  line L106 (82.9007, -12.2295) -> (82.186, -12.2295) projected
  line L107 (82.186, -12.2295) -> (82.186, -12.1542) projected
  line L108 (80.9972, -12.1614) -> (80.9972, -12.2295) projected
  line L109 (80.9972, -12.2295) -> (80.2921, -12.2295) projected
  line L110 (83.0928, -15.3584) -> (83.0928, -16.1801) projected
  line L111 (83.0928, -16.1801) -> (80.0928, -17.1939) projected
  line L112 (80.0928, -17.1939) -> (80.0928, -16.4183) projected
  line L113 (80.0928, -16.4183) -> (80.7054, -16.2311) projected
  line L114 (80.7054, -16.2311) -> (80.7054, -15.2879) projected
  line L115 (80.7054, -15.2879) -> (80.0928, -15.0982) projected
  line L116 (80.0928, -15.0982) -> (80.0928, -14.3446) projected
  line L117 (80.0928, -14.3446) -> (83.0928, -15.3584) projected
  line L118 (82.9007, -21.0107) -> (82.186, -21.0107) projected
  line L119 (82.186, -21.0107) -> (82.186, -20.9354) projected
  line L120 (80.9972, -20.9426) -> (80.9972, -21.0107) projected
  line L121 (80.9972, -21.0107) -> (80.2921, -21.0107) projected
  arc A4 (-66.3, -26) -> (-59.8, -32.5) centre (-59.8, -26) ccw projected
  line L122 (-59.8, -32.5) -> (89.8, -32.5) projected
  arc A5 (89.8, -32.5) -> (96.3, -26) centre (89.8, -26) ccw projected
  line L123 (96.3, -26) -> (96.3, 26) projected
  arc A6 (96.3, 26) -> (89.8, 32.5) centre (89.8, 26) ccw projected
  line L124 (89.8, 32.5) -> (-59.8, 32.5) projected
  arc A7 (-59.8, 32.5) -> (-66.3, 26) centre (-59.8, 26) ccw projected
  line L125 (-66.3, 26) -> (-66.3, -26) projected
  circle A8 centre (55.8, 9) radius 2.65 projected
  circle A9 centre (55.8, -6) radius 2.65 projected
  circle A10 centre (70.8, -16) radius 3.65 projected
  line L126 (-48.8, -20.25) -> (-48.8, 20.25) projected
  line L127 (-48.8, 20.25) -> (48.8, 20.25) projected
  line L128 (48.8, 20.25) -> (48.8, -20.25) projected
  line L129 (48.8, -20.25) -> (-48.8, -20.25) projected
  circle A11 centre (89.8, -26) radius 5.75 projected
  circle A12 centre (-59.8, 26) radius 5.75 projected
  circle A13 centre (46.5, 27.5) radius 4.5 projected
  circle A14 centre (-46.5, -27.5) radius 4.5 projected
  line L130 (76.95, -9.85) -> (64.65, -9.85)
  line L131 (64.65, -9.85) -> (64.65, -22.15)
  line L132 (64.65, -22.15) -> (76.95, -22.15)
  line L133 (76.95, -22.15) -> (76.95, -9.85)
  circle A15 centre (70.8, -16) radius 3.65 projected
  line L134 (76.95, -9.85) -> (64.65, -22.15) construction
  line L135 (64.65, -9.85) -> (76.95, -22.15) construction
  line L136 (78.95, -24.15) -> (62.65, -24.15)
  line L137 (62.65, -24.15) -> (62.65, -7.85)
  line L138 (62.65, -7.85) -> (78.95, -7.85)
  line L139 (78.95, -7.85) -> (78.95, -24.15)
  point P0 (0, 0)
  dimension "d98" = 12.3
  dimension "d99" = 12.3
  dimension "d100" = 2
  constraints: 20 end point, 4 parallel, 2 midpoint, 2 perpendicular, 1 horizontal, 81 other
  measures "d98" distance of L132.end L131.end
  measures "d99" distance of L131.end L130.end
  measures "d100" distance between parallel lines of L132 L136
extrude "Extrusión12" add sketch "Boceto19" along normal blind 5 contours L136 L137 L138 L139
chamfer "Chaflán4" distance 1 angle 45 3 edges at (62.65, 0, -16) (70.8, 0, -7.85) (70.8, 0, -24.15)
ref_plane "Plano de trabajo2" through (15, 0, 0) normal (-1, 0, 0) x (0, 1, 0)
